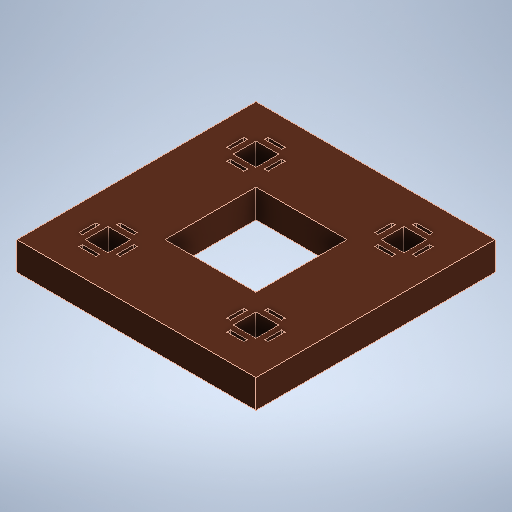
# Autodesk Inventor part: Box Of Fixation
Saved by Autodesk Inventor 2025.4 (Build 294407000, 407)
## iProperties
Created: 2026-05-09
Part Number: Box Of Fixation
Material: Generic
Document SubType Name: Modeling
Designer: lenovo
Density: 1 g/cm^3
Appearance: Default(1)
Author: lenovo
Autodesk Inventor part; units mm, degrees
ref_plane "YZ Plane" through (0, 0, 0) normal (1, 0, 0) x (0, 1, 0)
ref_plane "XZ Plane" through (0, 0, 0) normal (0, 1, 0) x (-1, 0, 0)
ref_plane "XY Plane" through (0, 0, 0) normal (0, 0, 1) x (1, 0, 0)
sketch "Sketch1" plane through (0, 0, 0) normal (0, 0, 1) x (1, 0, 0)
  line L0 (-105, 12.5) -> (105, 12.5)
  line L1 (105, 12.5) -> (105, -12.5)
  line L2 (105, -12.5) -> (-105, -12.5)
  line L3 (-105, -12.5) -> (-105, 12.5)
  line L4 (-105, 12.5) -> (105, -12.5) construction
  line L5 (105, 12.5) -> (-105, -12.5) construction
  point P0 (0, 0)
  dimension "d0" = 210
  dimension "d1" = 25
  constraints: 12 end point, 2 midpoint, 2 parallel, 1 horizontal, 1 perpendicular
  measures "d0" distance of L1.end L2.end
  measures "d1" distance of L0.end L1.end
extrude "Extrusion1" add sketch "Sketch1" along normal mid plane 210
sketch "Sketch2" plane through (-105, -12.5, 105) normal (0, -1, 0) x (1, 0, 0)
  line L0 (0, -210) -> (0, 0) projected
  line L1 (0, -40) -> (210, -40)
  line L2 (210, -210) -> (210, 0) projected
  line L3 (0, -170) -> (210, -170)
  line L4 (0, -105) -> (210, -105)
  line L5 (0, 0) -> (210, 0) projected
  line L6 (105, 0) -> (105, -210)
  line L7 (170, 0) -> (170, -210)
  line L8 (40, 0) -> (40, -210)
  line L9 (210, -210) -> (0, -210) projected
  line L10 (0, 0) -> (0, -210) projected
  line L11 (162.5, -21.92) -> (177.5, -21.92)
  line L12 (177.5, -21.92) -> (177.5, -25)
  line L13 (177.5, -25) -> (162.5, -25)
  line L14 (162.5, -25) -> (162.5, -21.92)
  line L15 (162.5, -21.92) -> (177.5, -25) construction
  line L16 (177.5, -21.92) -> (162.5, -25) construction
  line L17 (188.08, -32.5) -> (185, -32.5)
  line L18 (185, -32.5) -> (185, -47.5)
  line L19 (185, -47.5) -> (188.08, -47.5)
  line L20 (188.08, -47.5) -> (188.08, -32.5)
  line L21 (188.08, -32.5) -> (185, -47.5) construction
  line L22 (185, -32.5) -> (188.08, -47.5) construction
  line L23 (162.5, -58.08) -> (177.5, -58.08)
  line L24 (177.5, -58.08) -> (177.5, -55)
  line L25 (177.5, -55) -> (162.5, -55)
  line L26 (162.5, -55) -> (162.5, -58.08)
  line L27 (162.5, -58.08) -> (177.5, -55) construction
  line L28 (177.5, -58.08) -> (162.5, -55) construction
  line L29 (188.08, -47.5) -> (185, -47.5)
  line L30 (185, -47.5) -> (185, -32.5)
  line L31 (185, -32.5) -> (188.08, -32.5)
  line L32 (188.08, -32.5) -> (188.08, -47.5)
  line L33 (188.08, -47.5) -> (185, -32.5) construction
  line L34 (185, -47.5) -> (188.08, -32.5) construction
  line L35 (151.92, -32.5) -> (155, -32.5)
  line L36 (155, -32.5) -> (155, -47.5)
  line L37 (155, -47.5) -> (151.92, -47.5)
  line L38 (151.92, -47.5) -> (151.92, -32.5)
  line L39 (151.92, -32.5) -> (155, -47.5) construction
  line L40 (155, -32.5) -> (151.92, -47.5) construction
  line L41 (155, -32.5) -> (151.92, -32.5)
  line L42 (155, -47.5) -> (155, -32.5)
  line L43 (151.92, -32.5) -> (151.92, -47.5)
  line L44 (155, -47.5) -> (151.92, -32.5) construction
  line L45 (151.92, -47.5) -> (155, -47.5)
  line L46 (151.92, -47.5) -> (155, -32.5) construction
  line L47 (47.5, -21.92) -> (32.5, -21.92)
  line L48 (32.5, -21.92) -> (32.5, -25)
  line L49 (32.5, -25) -> (47.5, -25)
  line L50 (47.5, -25) -> (47.5, -21.92)
  line L51 (47.5, -21.92) -> (32.5, -25) construction
  line L52 (32.5, -21.92) -> (47.5, -25) construction
  line L53 (21.92, -32.5) -> (25, -32.5)
  line L54 (25, -32.5) -> (25, -47.5)
  line L55 (25, -47.5) -> (21.92, -47.5)
  line L56 (21.92, -47.5) -> (21.92, -32.5)
  line L57 (21.92, -32.5) -> (25, -47.5) construction
  line L58 (25, -32.5) -> (21.92, -47.5) construction
  line L59 (32.5, -55) -> (47.5, -55)
  line L60 (47.5, -58.08) -> (32.5, -58.08)
  line L61 (32.5, -58.08) -> (47.5, -55) construction
  line L62 (47.5, -58.08) -> (32.5, -55) construction
  line L63 (47.5, -55) -> (47.5, -58.08)
  line L64 (32.5, -58.08) -> (32.5, -55)
  line L65 (25, -32.5) -> (21.92, -32.5)
  line L66 (25, -47.5) -> (25, -32.5)
  line L67 (21.92, -32.5) -> (21.92, -47.5)
  line L68 (25, -47.5) -> (21.92, -32.5) construction
  line L69 (21.92, -47.5) -> (25, -47.5)
  line L70 (21.92, -47.5) -> (25, -32.5) construction
  line L71 (55, -32.5) -> (58.08, -32.5)
  line L72 (58.08, -32.5) -> (55, -32.5)
  line L73 (55, -47.5) -> (55, -32.5)
  line L74 (55, -32.5) -> (55, -47.5)
  line L75 (58.08, -47.5) -> (55, -47.5)
  line L76 (58.08, -32.5) -> (58.08, -47.5)
  line L77 (55, -47.5) -> (58.08, -32.5) construction
  line L78 (58.08, -47.5) -> (55, -32.5) construction
  line L79 (55, -47.5) -> (58.08, -47.5)
  line L80 (58.08, -47.5) -> (58.08, -32.5)
  line L81 (55, -32.5) -> (58.08, -47.5) construction
  line L82 (58.08, -32.5) -> (55, -47.5) construction
  line L83 (162.5, -188.08) -> (177.5, -188.08)
  line L84 (177.5, -188.08) -> (177.5, -185)
  line L85 (177.5, -185) -> (162.5, -185)
  line L86 (162.5, -185) -> (162.5, -188.08)
  line L87 (162.5, -188.08) -> (177.5, -185) construction
  line L88 (177.5, -188.08) -> (162.5, -185) construction
  line L89 (188.08, -177.5) -> (185, -177.5)
  line L90 (185, -177.5) -> (185, -162.5)
  line L91 (185, -162.5) -> (188.08, -162.5)
  line L92 (188.08, -162.5) -> (188.08, -177.5)
  line L93 (188.08, -177.5) -> (185, -162.5) construction
  line L94 (185, -177.5) -> (188.08, -162.5) construction
  line L95 (177.5, -155) -> (162.5, -155)
  line L96 (162.5, -151.92) -> (177.5, -151.92)
  line L97 (177.5, -151.92) -> (162.5, -155) construction
  line L98 (162.5, -151.92) -> (177.5, -155) construction
  line L99 (162.5, -155) -> (162.5, -151.92)
  line L100 (177.5, -151.92) -> (177.5, -155)
  line L101 (185, -177.5) -> (188.08, -177.5)
  line L102 (185, -162.5) -> (185, -177.5)
  line L103 (188.08, -177.5) -> (188.08, -162.5)
  line L104 (185, -162.5) -> (188.08, -177.5) construction
  line L105 (188.08, -162.5) -> (185, -162.5)
  line L106 (188.08, -162.5) -> (185, -177.5) construction
  line L107 (155, -177.5) -> (151.92, -177.5)
  line L108 (151.92, -177.5) -> (155, -177.5)
  line L109 (155, -162.5) -> (155, -177.5)
  line L110 (155, -177.5) -> (155, -162.5)
  line L111 (151.92, -162.5) -> (155, -162.5)
  line L112 (151.92, -177.5) -> (151.92, -162.5)
  line L113 (155, -162.5) -> (151.92, -177.5) construction
  line L114 (151.92, -162.5) -> (155, -177.5) construction
  line L115 (155, -162.5) -> (151.92, -162.5)
  line L116 (151.92, -162.5) -> (151.92, -177.5)
  line L117 (155, -177.5) -> (151.92, -162.5) construction
  line L118 (151.92, -177.5) -> (155, -162.5) construction
  line L119 (55, -177.5) -> (58.08, -177.5)
  line L120 (58.08, -177.5) -> (58.08, -162.5)
  line L121 (55, -162.5) -> (58.08, -177.5) construction
  line L122 (58.08, -162.5) -> (55, -177.5) construction
  line L123 (58.08, -177.5) -> (55, -177.5)
  line L124 (58.08, -162.5) -> (58.08, -177.5)
  line L125 (55, -177.5) -> (58.08, -162.5) construction
  line L126 (58.08, -177.5) -> (55, -162.5) construction
  line L127 (58.08, -162.5) -> (55, -162.5)
  line L128 (55, -162.5) -> (58.08, -162.5)
  line L129 (25, -162.5) -> (21.92, -162.5)
  line L130 (21.92, -162.5) -> (25, -162.5)
  line L131 (25, -177.5) -> (25, -162.5)
  line L132 (25, -162.5) -> (25, -177.5)
  line L133 (21.92, -162.5) -> (21.92, -177.5)
  line L134 (25, -177.5) -> (21.92, -162.5) construction
  line L135 (21.92, -177.5) -> (25, -162.5) construction
  line L136 (21.92, -177.5) -> (25, -177.5)
  line L137 (21.92, -162.5) -> (25, -177.5) construction
  line L138 (21.92, -177.5) -> (21.92, -162.5)
  line L139 (25, -177.5) -> (21.92, -177.5)
  line L140 (25, -162.5) -> (21.92, -177.5) construction
  line L141 (47.5, -188.08) -> (32.5, -188.08)
  line L142 (32.5, -188.08) -> (32.5, -185)
  line L143 (32.5, -185) -> (47.5, -185)
  line L144 (47.5, -185) -> (47.5, -188.08)
  line L145 (47.5, -188.08) -> (32.5, -185) construction
  line L146 (32.5, -188.08) -> (47.5, -185) construction
  line L147 (55, -162.5) -> (55, -177.5)
  line L148 (55, -177.5) -> (55, -162.5)
  line L149 (32.5, -151.92) -> (32.5, -155)
  line L150 (32.5, -155) -> (47.5, -155)
  line L151 (32.5, -151.92) -> (47.5, -155) construction
  line L152 (47.5, -151.92) -> (32.5, -155) construction
  line L153 (47.5, -155) -> (47.5, -151.92)
  line L154 (47.5, -151.92) -> (32.5, -151.92)
  line L155 (160, -30) -> (180, -30)
  line L156 (180, -30) -> (180, -50)
  line L157 (180, -50) -> (160, -50)
  line L158 (160, -50) -> (160, -30)
  line L159 (160, -30) -> (180, -50) construction
  line L160 (180, -30) -> (160, -50) construction
  line L161 (30, -50) -> (50, -50)
  line L162 (50, -50) -> (50, -30)
  line L163 (50, -30) -> (30, -30)
  line L164 (30, -30) -> (30, -50)
  line L165 (30, -50) -> (50, -30) construction
  line L166 (50, -50) -> (30, -30) construction
  line L167 (30, -160) -> (50, -160)
  line L168 (50, -160) -> (50, -180)
  line L169 (50, -180) -> (30, -180)
  line L170 (30, -180) -> (30, -160)
  line L171 (30, -160) -> (50, -180) construction
  line L172 (50, -160) -> (30, -180) construction
  line L173 (160, -160) -> (180, -160)
  line L174 (180, -160) -> (180, -180)
  line L175 (180, -180) -> (160, -180)
  line L176 (160, -180) -> (160, -160)
  line L177 (160, -160) -> (180, -180) construction
  line L178 (180, -160) -> (160, -180) construction
  point P0 (105, -105)
  point P1 (170, -23.46)
  point P2 (186.54, -40)
  point P3 (170, -56.54)
  point P4 (153.46, -40)
  point P5 (40, -23.46)
  point P6 (23.46, -40)
  point P7 (40, -56.54)
  point P8 (56.54, -40)
  point P9 (170, -186.54)
  point P10 (186.54, -170)
  point P11 (170, -153.46)
  point P12 (153.46, -170)
  point P13 (56.54, -170)
  point P14 (23.46, -170)
  point P15 (40, -186.54)
  point P16 (40, -153.46)
  point P17 (170, -40)
  point P18 (40, -40)
  point P19 (40, -170)
  point P20 (170, -170)
  dimension "d4" = 40
  dimension "d5" = 40
  dimension "d8" = 15
  dimension "d9" = 3.08
  dimension "d10" = 30
  dimension "d11" = 15
  dimension "d12" = 30
  dimension "d13" = 3.08
  dimension "d20" = 20
  dimension "d21" = 20
  dimension "d22" = 20
  dimension "d23" = 20
  dimension "d24" = 20
  dimension "d25" = 20
  dimension "d26" = 20
  dimension "d27" = 20
  constraints: 348 end point, 102 symmetric about line, 18 point on line, 16 midpoint, 12 parallel, 8 horizontal, 8 perpendicular, 1 vertical, 2 other
  measures "d4" distance between parallel lines of L2 L7
  measures "d5" distance between parallel lines of L5 L1
  measures "d8" distance of L12.end L13.end
  measures "d9" distance of L11.end L12.end
  measures "d10" diameter of L13 L1
  measures "d11" distance between parallel lines of L17 L19
  measures "d12" diameter of L18 L7
  measures "d13" distance of L18.end L19.end
  measures "d20" distance of L156.end L157.end
  measures "d21" distance of L155.end L156.end
  measures "d22" distance of L163.end L162.end
  measures "d23" distance of L162.end L161.end
  measures "d24" distance of L168.end L169.end
  measures "d25" distance of L167.end L168.end
  measures "d26" distance of L174.end L175.end
  measures "d27" distance of L173.end L174.end
extrude "Extrusion2" cut sketch "Sketch2" against normal through all contours L133 L129 L131 L3 | L3 L131 L136 L133 | L141 L142 L143 L8 | L8 L143 L144 L141 | L56 L53 L54 L1 | L1 L54 L55 L56 | L60 L64 L59 L8 | L8 L59 L63 L60 | L154 L153 L150 L8 | L8 L150 L149 L154 | L170 L167 L8 L3 | L3 L8 L169 L170 | L8 L3 L168 L169 | L120 L119 L147 L3 | L3 L147 L127 L120 | L112 L111 L109 L3 | L3 L109 L107 L112 | L83 L86 L85 L7 | L7 L85 L84 L83 | L8 L167 L168 L3 | L47 L50 L49 L8 | L8 L49 L48 L47 | L164 L163 L8 L1 | L1 L8 L161 L164 | L23 L26 L25 L7 | L7 L25 L24 L23 | L96 L100 L95 L7 | L7 L95 L99 L96 | L76 L75 L73 L1 | L1 L73 L71 L76 | L38 L35 L36 L1 | L1 L36 L37 L38 | L8 L1 L162 L161 | L176 L173 L7 L3 | L3 L7 L175 L176 | L7 L3 L174 L175 | L92 L89 L90 L3 | L3 L90 L91 L92 | L8 L163 L162 L1 | L7 L173 L174 L3 | L11 L12 L13 L7 | L7 L13 L14 L11 | L20 L19 L18 L1 | L1 L18 L17 L20 | L157 L158 L1 L7 | L7 L1 L156 L157 | L158 L155 L7 L1 | L7 L155 L156 L1
sketch "Sketch3" plane through (-105, 12.5, 105) normal (0, 1, 0) x (1, 0, 0)
  line L0 (65, 65) -> (145, 65)
  line L1 (145, 65) -> (145, 145)
  line L2 (145, 145) -> (65, 145)
  line L3 (65, 145) -> (65, 65)
  line L4 (65, 65) -> (145, 145) construction
  line L5 (145, 65) -> (65, 145) construction
  point P0 (105, 105)
  dimension "d16" = 80
  dimension "d17" = 80
  constraints: 12 end point, 2 midpoint, 2 parallel, 1 horizontal, 1 perpendicular
  measures "d16" distance of L2.end L1.end
  measures "d17" distance of L1.end L0.end
extrude "Extrusion3" cut sketch "Sketch3" against normal through all
equation "\"d5\" = d4"
equation "\"d12\" = d10"
equation "\"d13\" = d9"
body "Solid1"
